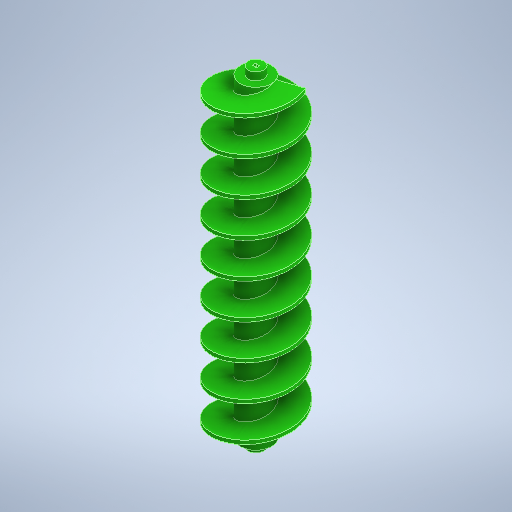
# Autodesk Inventor part: Lifting mechanism
Saved by Autodesk Inventor 2025.4 (Build 294407000, 407)
## iProperties
Created: 2026-03-02
Part Number: Lifting mechanism
Material: Generic
Document SubType Name: Modeling
Designer: abdo2
Density: 1 g/cm^3
Appearance: Default(1)
Author: abdo2
Autodesk Inventor part; units mm, degrees
ref_plane "YZ Plane" through (0, 0, 0) normal (1, 0, 0) x (0, 1, 0)
ref_plane "XZ Plane" through (0, 0, 0) normal (0, 1, 0) x (-1, 0, 0)
ref_plane "XY Plane" through (0, 0, 0) normal (0, 0, 1) x (1, 0, 0)
sketch "Sketch1" plane through (0, 0, 0) normal (0, 1, 0) x (-1, 0, 0)
  circle A0 centre (0, 0) radius 20
  dimension "d0" = 40
  constraints: 1 centre point, 1 coincident
  measures "d0" diameter of A0
extrude "Extrusion1" add sketch "Sketch1" along normal mid plane 400
sketch "Sketch2" plane through (0, 0, 0) normal (1, 0, 0) x (0, 1, 0)
  line L0 (-200, 20) -> (-200, -20) projected
  line L1 (-200, -20) -> (-200, -50)
  line L2 (-200, -50) -> (-195, -50)
  line L3 (-195, -50) -> (-195, -20)
  line L4 (-195, -20) -> (-200, -20)
  line L5 (-200, -20) -> (200, -20) projected
  line L6 (-264, 0) -> (283, 0) construction
  point P0 (0, 0)
  dimension "d3" = 30
  dimension "d4" = 5
  constraints: 10 end point, 2 horizontal, 1 collinear, 1 perpendicular, 1 vertical
  measures "d3" distance of L0.end L1.end
  measures "d4" distance of L1.end L2.end
coil "Coil1" sketch "Sketch2" operation add axis through (0, -264, 0) along (0, 1, 0) pitch 45 turns 8.8 hand right
sketch "Sketch3" plane through (0, 200, 0) normal (0, 1, 0) x (0.2419, 0, 0.9703)
  point P0 (0, 0)
sketch "Sketch4" plane through (0, 200, 0) normal (0, 1, 0) x (0.2419, 0, 0.9703)
  circle A0 centre (0, 0) radius 10
  dimension "d13" = 20
  constraints: 1 centre point, 1 coincident
  measures "d13" diameter of A0
extrude "Extrusion2" add sketch "Sketch4" along normal blind 10
sketch "Sketch5" plane through (0, 210, 0) normal (0, 1, 0) x (1, 0, 0)
  circle A0 centre (0, 0) radius 2.75
  line L0 (-1.9391, 1.95) -> (1.9391, 1.95)
  line L1 (-1.9391, -1.95) -> (1.9391, -1.95)
  dimension "d16" = 5.5
  dimension "d17" = 1.95
  dimension "d18" = 3.9
  constraints: 4 end point, 4 point on circle, 2 horizontal, 1 centre point, 1 coincident
  measures "d16" diameter of A0
  measures "d17" distance from line of point (0, 0) L0
  measures "d18" distance between parallel lines of L0 L1
extrude "Extrusion3" cut sketch "Sketch5" against normal blind 10 contours A0 L1 L0
sketch "Sketch6" plane through (0, -200, 0) normal (0, -1, 0) x (1, 0, 0)
  circle A0 centre (0, 0) radius 10
  dimension "d21" = 20
  constraints: 1 centre point, 1 coincident
  measures "d21" diameter of A0
extrude "Extrusion4" add sketch "Sketch6" along normal blind 10
sketch "Sketch7" plane through (0, -210, 0) normal (0, -1, 0) x (1, 0, 0)
  circle A0 centre (0, 0) radius 2.75
  line L0 (1.9391, -1.95) -> (-1.9391, -1.95)
  line L1 (1.9391, 1.95) -> (-1.9391, 1.95)
  line L2 (1.9391, 1.95) -> (-1.9391, 1.95) projected
  dimension "d24" = 5.5
  dimension "d25" = 1.95
  dimension "d26" = 3.9
  constraints: 4 end point, 4 point on circle, 1 centre point, 1 coincident, 1 collinear, 1 horizontal
  measures "d24" diameter of A0
  measures "d25" distance from line of point (0, 0) L0
  measures "d26" distance between parallel lines of L0 L1
extrude "Extrusion5" cut sketch "Sketch7" against normal blind 10 contours A0 L0 L1
body "Solid1"
